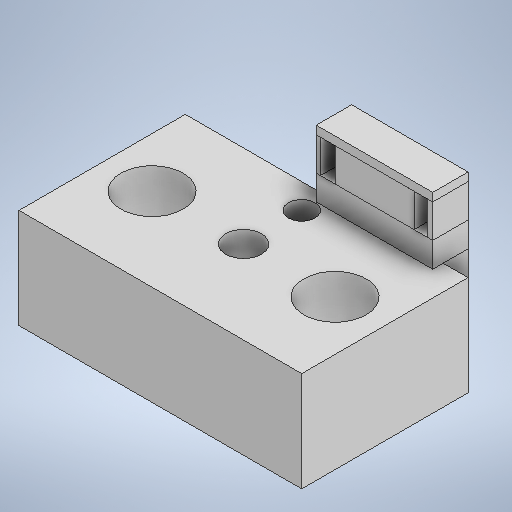
# Autodesk Inventor part: Taster_Schlitten_M8
Saved by Autodesk Inventor 2025 (Build 290162000, 162)
## iProperties
Created: 2026-07-13
Part Number: Taster_Schlitten_M8
Material: Generisch
Document SubType Name: Modeling
Designer: wavid
Mass: 59.5301 g
Surface Area: 181.552 cm^2
Volume: 59.5301 cm^3
Density: 1 g/cm^3
Appearance: Vorgabe
Author: wavid
Autodesk Inventor part; units mm, degrees
sketch "Skizze1" plane through (0, 0, 0) normal (0, 0, 1) x (1, 0, 0)
  line L0 (-34, -20) -> (34, -20)
  line L1 (34, -20) -> (34, 20)
  line L2 (34, 20) -> (-34, 20)
  line L3 (-34, 20) -> (-34, -20)
  constraints: 8 end point, 2 parallel, 1 horizontal, 1 perpendicular
extrude "Extrusion1" add sketch "Skizze1" along normal blind 24
sketch "Skizze2" plane through (0, 0, 0) normal (0, 0, 1) x (1, 0, 0)
  line L0 (0, 20) -> (28, 20)
  line L1 (28, 20) -> (28, 26)
  line L2 (28, 26) -> (0, 26)
  line L3 (0, 26) -> (0, 20)
  constraints: 8 end point, 2 parallel, 1 horizontal, 1 perpendicular
extrude "Extrusion2" add sketch "Skizze2" along normal blind 24 separate body
ref_plane "Arbeitsebene1" through (0, 0, 24) normal (0, 0, 1) x (1, 0, 0)
sketch "Skizze3" plane through (0, 0, 24) normal (0, 0, 1) x (1, 0, 0)
  line L0 (0, 17.5) -> (28, 17.5)
  line L1 (28, 17.5) -> (28, 26)
  line L2 (28, 26) -> (0, 26)
  line L3 (0, 26) -> (0, 17.5)
  constraints: 8 end point, 2 parallel, 1 horizontal, 1 perpendicular
extrude "Extrusion3" add sketch "Skizze3" along normal blind 6 separate body
ref_plane "Arbeitsebene2" through (0, 0, 30) normal (0, 0, 1) x (1, 0, 0)
sketch "Skizze4" plane through (0, 0, 30) normal (0, 0, 1) x (1, 0, 0)
  line L0 (0, 17.5) -> (1, 17.5)
  line L1 (1, 17.5) -> (1, 26)
  line L2 (1, 26) -> (0, 26)
  line L3 (0, 26) -> (0, 17.5)
  constraints: 8 end point, 2 parallel, 1 horizontal, 1 perpendicular
extrude "Extrusion4" add sketch "Skizze4" along normal blind 8 separate body
sketch "Skizze5" plane through (0, 0, 30) normal (0, 0, 1) x (1, 0, 0)
  line L0 (4.5, 17.5) -> (23.5, 17.5)
  line L1 (23.5, 17.5) -> (23.5, 26)
  line L2 (23.5, 26) -> (4.5, 26)
  line L3 (4.5, 26) -> (4.5, 17.5)
  constraints: 8 end point, 2 parallel, 1 horizontal, 1 perpendicular
extrude "Extrusion5" add sketch "Skizze5" along normal blind 8 separate body
sketch "Skizze6" plane through (0, 0, 30) normal (0, 0, 1) x (1, 0, 0)
  line L0 (26.7, 17.5) -> (28, 17.5)
  line L1 (28, 17.5) -> (28, 26)
  line L2 (28, 26) -> (26.7, 26)
  line L3 (26.7, 26) -> (26.7, 17.5)
  constraints: 8 end point, 2 parallel, 1 horizontal, 1 perpendicular
extrude "Extrusion6" add sketch "Skizze6" along normal blind 8 separate body
ref_plane "Arbeitsebene3" through (0, 0, 38) normal (0, 0, 1) x (1, 0, 0)
sketch "Skizze7" plane through (0, 0, 38) normal (0, 0, 1) x (1, 0, 0)
  line L0 (0, 17.5) -> (28, 17.5)
  line L1 (28, 17.5) -> (28, 26)
  line L2 (28, 26) -> (0, 26)
  line L3 (0, 26) -> (0, 17.5)
  constraints: 8 end point, 2 parallel, 1 horizontal, 1 perpendicular
extrude "Extrusion7" add sketch "Skizze7" along normal blind 2 separate body
sketch "Skizze8" plane through (0, 0, 24) normal (0, 0, 1) x (1, 0, 0)
  circle A0 centre (-22, 0) radius 7.5
  constraints: 1 centre point
extrude "Extrusion8" cut sketch "Skizze8" against normal blind 24.2 bodies 1
sketch "Skizze9" plane through (0, 0, 24) normal (0, 0, 1) x (1, 0, 0)
  circle A0 centre (22, 0) radius 7.5
  constraints: 1 centre point
extrude "Extrusion9" cut sketch "Skizze9" against normal blind 24.2 bodies 1
sketch "Skizze10" plane through (0, 0, 24) normal (0, 0, 1) x (1, 0, 0)
  circle A0 centre (0, 0) radius 4.3
  constraints: 1 centre point
extrude "Extrusion10" cut sketch "Skizze10" against normal blind 24.2 bodies 1
sketch "Skizze11" plane through (0, 0, 24) normal (0, 0, 1) x (1, 0, 0)
  circle A0 centre (0, 14) radius 3.2
  constraints: 1 centre point
extrude "Extrusion11" cut sketch "Skizze11" against normal blind 24.2 bodies 1
sketch "Skizze12" plane through (0, 0, 0) normal (0, 0, 1) x (1, 0, 0)
  line L0 (-6.7, -7.8) -> (6.7, -7.8)
  line L1 (6.7, -7.8) -> (6.7, 7.8)
  line L2 (6.7, 7.8) -> (-6.7, 7.8)
  line L3 (-6.7, 7.8) -> (-6.7, -7.8)
  constraints: 8 end point, 2 parallel, 1 horizontal, 1 perpendicular
extrude "Extrusion12" cut sketch "Skizze12" along normal blind 7 bodies 1
sketch "Skizze13" plane through (0, 0, 0) normal (0, 0, 1) x (1, 0, 0)
  circle A0 centre (0, 14) radius 6.5
  constraints: 1 centre point
extrude "Extrusion13" cut sketch "Skizze13" along normal blind 14 bodies 1
sketch "Skizze14" plane through (0, 0, 0) normal (0, 0, 1) x (1, 0, 0)
  circle A0 centre (-9, 14) radius 1
  constraints: 1 centre point
extrude "Extrusion14" cut sketch "Skizze14" along normal blind 8 bodies 1
sketch "Skizze15" plane through (0, 0, 0) normal (0, 0, 1) x (1, 0, 0)
  circle A0 centre (9, 14) radius 1
  constraints: 1 centre point
extrude "Extrusion15" cut sketch "Skizze15" along normal blind 8 bodies 1
